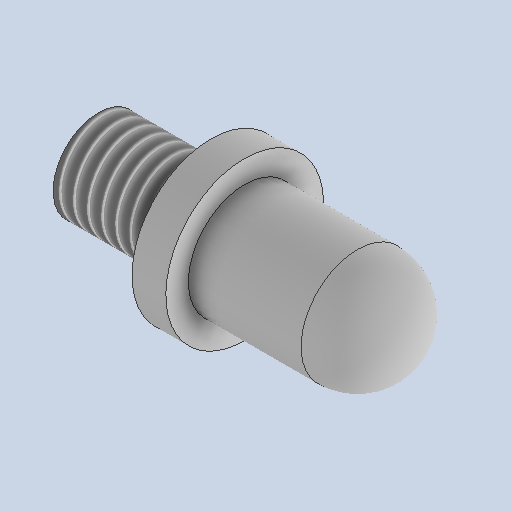
# Autodesk Inventor part: 1156
Saved by Autodesk Inventor 2025.1 (Build 291241000, 241)
## iProperties
Created: 2024-06-07
Part Number: 1156
Material: Generisch
Document SubType Name: Modeling
Designer: ffogue
Density: 1 g/cm^3
Appearance: Vorgabe
Author: ffogue
Autodesk Inventor part; units mm, degrees
ref_plane "YZ Plane" through (0, 0, 0) normal (1, 0, 0) x (0, 1, 0)
ref_plane "XZ Plane" through (0, 0, 0) normal (0, 1, 0) x (-1, 0, 0)
ref_plane "XY Plane" through (0, 0, 0) normal (0, 0, 1) x (1, 0, 0)
sketch "Skizze1" plane through (0, 0, 0) normal (0, 1, 0) x (-1, 0, 0)
  line L0 (0, 0) -> (0, 4)
  line L1 (0, 4) -> (-10, 4)
  line L2 (-10, 4) -> (-10, 7)
  line L3 (-10, 7) -> (-13, 7)
  line L4 (-13, 7) -> (-13, 5)
  line L5 (-13, 5) -> (-23, 5)
  arc A0 (-23, 5) -> (-28, 0) centre (-23, 0) ccw
  line L6 (0, 0) -> (-28, 0)
  dimension "d0" = 3
  dimension "d1" = 10
  dimension "d2" = 15
  dimension "d3" = 14
  dimension "d4" = 8
  dimension "d5" = 10
  constraints: 14 end point, 5 perpendicular, 2 point on circle, 1 centre point, 1 horizontal, 1 horizontal alignment, 1 tangent, 1 vertical
  measures "d0" distance of L2.end L3.end
  measures "d1" distance of L0.end L1.end
  measures "d2" horizontal distance of L6.end L3.end
  measures "d3" diameter of L3 L6
  measures "d4" diameter of L1 L6
  measures "d5" diameter of L5 L6
revolve "Umdrehung1" add sketch "Skizze1" angle 360 about axis through (0, 0, 0) along (1, 0, 0)
thread "Gewinde1" size "M8x1.25" class "6g" standard "ISO Metric profile" length 10
sketch "Skizze2" plane through (0, 0, 0) normal (-1, 0, 0) x (0, 0, 1)
  circle A0 centre (0, 0) radius 4 projected
  point P0 (0, 0)
  constraints: 1 coincident
hole "Bohrung1" at (0, 0, 0) direction (1, 0, 0) diameter 5 depth 25
